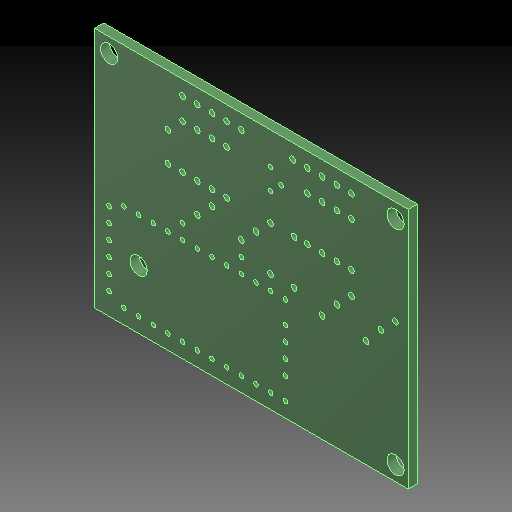
# Autodesk Inventor part: BATTERIES_CONTROLLER.brdКонтур
Saved by Autodesk Inventor 2020 (Build 240168000, 168)
## iProperties
Created: 2021-08-07
Part Number: BATTERIES_CONTROLLER.brdКонтур
Material: Типовые
Document SubType Name: Modeling
Designer: Петров Иван
Mass: 3.50945 g
Surface Area: 51.231 cm^2
Volume: 3.50945 cm^3
Density: 1 g/cm^3
Appearance: Контур панели
Author: Петров Иван
Autodesk Inventor part; units mm, degrees
ref_plane "YZ Plane" through (0, 0, 0) normal (1, 0, 0) x (0, 1, 0)
ref_plane "XZ Plane" through (0, 0, 0) normal (0, 1, 0) x (-1, 0, 0)
ref_plane "XY Plane" through (0, 0, 0) normal (0, 0, 1) x (1, 0, 0)
sketch "Эскиз1" plane through (0, 0, 0) normal (0, 0, 1) x (1, 0, 0)
  line L0 (0, 0) -> (54.28, 0)
  line L1 (54.28, 0) -> (54.28, 41.9)
  line L2 (54.28, 41.9) -> (0, 41.9)
  line L3 (0, 41.9) -> (0, 0)
  circle A0 centre (15.24, 39.37) radius 0.5
  circle A1 centre (17.78, 39.37) radius 0.5
  circle A2 centre (20.32, 39.37) radius 0.5
  circle A3 centre (22.86, 39.37) radius 0.5
  circle A4 centre (25.4, 39.37) radius 0.5
  circle A5 centre (34.29, 39.37) radius 0.5
  circle A6 centre (36.83, 39.37) radius 0.5
  circle A7 centre (39.37, 39.37) radius 0.5
  circle A8 centre (41.91, 39.37) radius 0.5
  circle A9 centre (44.45, 39.37) radius 0.5
  circle A10 centre (30.48, 32.75) radius 0.405
  circle A11 centre (32.28, 34.54) radius 0.405
  circle A12 centre (30.48, 36.34) radius 0.405
  circle A13 centre (44.45, 24) radius 0.5
  circle A14 centre (52.07, 24) radius 0.5
  circle A15 centre (41.91, 21.46) radius 0.5
  circle A16 centre (49.53, 21.46) radius 0.5
  circle A17 centre (39.37, 18.54) radius 0.5
  circle A18 centre (46.99, 18.54) radius 0.5
  circle A19 centre (34.54, 20.32) radius 0.5
  circle A20 centre (34.54, 27.94) radius 0.5
  circle A21 centre (44.45, 35.56) radius 0.5
  circle A22 centre (44.45, 27.94) radius 0.5
  circle A23 centre (41.91, 35.56) radius 0.5
  circle A24 centre (41.91, 27.94) radius 0.5
  circle A25 centre (39.37, 35.56) radius 0.5
  circle A26 centre (39.37, 27.94) radius 0.5
  circle A27 centre (36.83, 35.56) radius 0.5
  circle A28 centre (36.83, 27.94) radius 0.5
  circle A29 centre (30.48, 27.94) radius 0.5
  circle A30 centre (30.48, 20.32) radius 0.5
  circle A31 centre (20.32, 25.4) radius 0.5
  circle A32 centre (27.94, 25.4) radius 0.5
  circle A33 centre (17.78, 22.86) radius 0.5
  circle A34 centre (25.4, 22.86) radius 0.5
  circle A35 centre (15.24, 20.32) radius 0.405
  circle A36 centre (25.4, 20.32) radius 0.405
  circle A37 centre (22.86, 35.56) radius 0.5
  circle A38 centre (22.86, 27.94) radius 0.5
  circle A39 centre (20.32, 35.56) radius 0.5
  circle A40 centre (20.32, 27.94) radius 0.5
  circle A41 centre (17.78, 35.56) radius 0.5
  circle A42 centre (17.78, 27.94) radius 0.5
  circle A43 centre (15.24, 35.56) radius 0.5
  circle A44 centre (15.24, 27.94) radius 0.5
  circle A45 centre (22.86, 17.78) radius 0.4
  circle A46 centre (20.32, 17.78) radius 0.4
  circle A47 centre (17.78, 17.78) radius 0.4
  circle A48 centre (15.24, 17.78) radius 0.4
  circle A49 centre (33.02, 6.35) radius 0.4
  circle A50 centre (33.02, 8.89) radius 0.4
  circle A51 centre (33.02, 11.43) radius 0.4
  circle A52 centre (33.02, 13.97) radius 0.4
  circle A53 centre (15.24, 2.54) radius 0.4
  circle A54 centre (17.78, 2.54) radius 0.4
  circle A55 centre (20.32, 2.54) radius 0.4
  circle A56 centre (22.86, 2.54) radius 0.4
  circle A57 centre (25.4, 2.54) radius 0.4
  circle A58 centre (27.94, 2.54) radius 0.4
  circle A59 centre (30.48, 2.54) radius 0.4
  circle A60 centre (33.02, 2.54) radius 0.4
  circle A61 centre (33.02, 17.78) radius 0.4
  circle A62 centre (30.48, 17.78) radius 0.4
  circle A63 centre (27.94, 17.78) radius 0.4
  circle A64 centre (25.4, 17.78) radius 0.4
  circle A65 centre (2.54, 16.51) radius 0.4
  circle A66 centre (7.62, 17.78) radius 0.4
  circle A67 centre (12.7, 2.54) radius 0.4
  circle A68 centre (2.54, 3.81) radius 0.4
  circle A69 centre (2.54, 6.35) radius 0.4
  circle A70 centre (5.08, 17.78) radius 0.4
  circle A71 centre (10.16, 17.78) radius 0.4
  circle A72 centre (10.16, 2.54) radius 0.4
  circle A73 centre (7.62, 2.54) radius 0.4
  circle A74 centre (2.54, 11.43) radius 0.4
  circle A75 centre (5.08, 2.54) radius 0.4
  circle A76 centre (2.54, 13.97) radius 0.4
  circle A77 centre (12.7, 17.78) radius 0.4
  circle A78 centre (2.54, 8.89) radius 0.4
  circle A79 centre (2.54, 39.37) radius 1.5
  circle A80 centre (52.07, 39.37) radius 1.5
  circle A81 centre (52.07, 2.54) radius 1.5
  circle A82 centre (7.62, 10.16) radius 1.5
  circle A83 centre (12.7, 33.02) radius 0.5
  circle A84 centre (12.7, 27.94) radius 0.5
  constraints: 85 centre point, 8 end point
extrude "BATTERIES_CONTROLLER.brdКонтур" add sketch "Эскиз1" along normal blind 1.6
